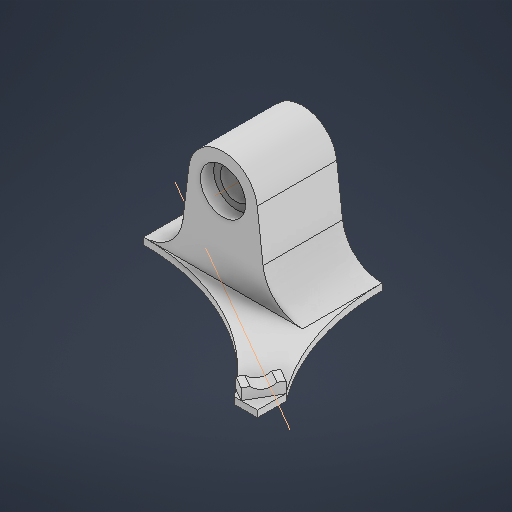
# Autodesk Inventor part: Support
Saved by Autodesk Inventor 2025.3 (Build 293356030, 356C)
## iProperties
Created: 2025-09-22
Part Number: Support
Material: Generic
Document SubType Name: Modeling
Designer: yo
Density: 1 g/cm^3
Appearance: Default
Author: yo
Autodesk Inventor part; units mm, degrees
ref_plane "YZ Plane" through (0, 0, 0) normal (1, 0, 0) x (0, 1, 0)
ref_plane "XZ Plane" through (0, 0, 0) normal (0, 1, 0) x (-1, 0, 0)
sketch "Sketch1" plane through (0, 0, 0) normal (0, 0, 1) x (1, 0, 0)
  circle A0 centre (0, 30) radius 8.525
  circle A1 centre (0, 30) radius 6
  arc A2 (-30, 0) -> (-15.1068, 13.2135) centre (-30, 15) ccw
  arc A3 (15.1068, 13.2135) -> (30, 0) centre (30, 15) ccw
  arc A4 (12.9075, 31.5483) -> (-12.9075, 31.5483) centre (0, 30) ccw
  line L0 (-12.9075, 31.5483) -> (-15.1068, 13.2135)
  line L1 (12.9075, 31.5483) -> (15.1068, 13.2135)
  line L2 (30, 0) -> (-30, 0)
  line L3 (-30, 0) -> (-30, -2.5)
  line L4 (-30, -2.5) -> (30, -2.5)
  line L5 (30, -2.5) -> (30, 0)
  point P0 (0, 0)
  point P1 (0, 0)
  dimension "d2" = 17.05
  dimension "d3" = 12
  dimension "d9" = 30
  dimension "d12" = 13
  dimension "d15" = 15
  dimension "d16" = 60
  dimension "d17" = 2.5
  constraints: 12 end point, 6 point on circle, 5 centre point, 5 tangent, 3 coincident, 2 horizontal alignment, 2 perpendicular, 2 vertical alignment, 1 equal length, 1 equal radius, 1 horizontal, 1 midpoint, 1 vertical
  measures "d2" diameter of A0
  measures "d3" diameter of A1
  measures "d9" distance of point (0, 0) A0.centre
  measures "d12" radius of A4
  measures "d15" radius of A2
  measures "d16" distance of L3.end L4.end
  measures "d17" distance of L2.end L3.end
extrude "Extrusion3" add sketch "Sketch1" along normal mid plane 30 contours A2 L0 A4 L1 A3 L2
extrude "Extrusion4" add sketch "Sketch1" along normal mid plane 20 contours A0
extrude "Extrusion5" add sketch "Sketch1" against normal blind 15 contours L2 L5 L4 L3
extrude "Extrusion6" add sketch "Sketch1" along normal blind 50 contours L2 L5 L4 L3
ref_plane "Work Plane1" through (30, -2.5, 50) normal (0.866, 0, 0.5) x (0, 1, 0)
ref_plane "Work Plane3" through (36.4952, -2.5, 53.75) normal (0.866, 0, 0.5) x (0, 1, 0)
sketch "Sketch5" plane through (36.4952, -2.5, 53.75) normal (0.866, 0, 0.5) x (0, 1, 0)
  line L0 (2.5, -30.3109) -> (2.5, -18.3109) construction
  circle A0 centre (10.5, -12.1087) radius 5.35
  circle A1 centre (10.5, -12.1087) radius 7.3 construction
  line L1 (2.5, -18.3109) -> (6.65, -18.3109)
  line L2 (6.65, -18.3109) -> (6.65, -5.9065)
  line L3 (6.65, -5.9065) -> (2.5, -5.9065)
  line L4 (2.5, -5.9065) -> (2.5, -18.3109)
  point P0 (6.65, -15.8235)
  point P1 (6.65, -8.3938)
  dimension "d46" = 12
  dimension "d47" = 10.7
  dimension "d48" = 14.6
  dimension "d49" = 8
  dimension "d51" = 1.5
  constraints: 10 end point, 2 centre point, 2 parallel, 2 point on circle, 1 coincident, 1 horizontal, 1 perpendicular, 1 vertical
  measures "d46" distance of L0.start L0.end
  measures "d47" diameter of A0
  measures "d48" diameter of A1
  measures "d49" distance from line of L4 A0.centre
  measures "d51" distance edge to line of A0 L2
extrude "Extrusion9" add sketch "Sketch5" along normal mid plane 5.5 contours A0 L2 L1 L4 L3
sketch "Sketch6" plane through (30, -2.5, -15) normal (1, 0, 0) x (0, 0, -1)
  line L0 (0, 0) -> (-65, 0) projected
  line L1 (0, 2.5) -> (0, 0) projected
  line L2 (0, 2.5) -> (-30, 2.5) projected
  line L3 (-30, 2.5) -> (-65, 2.5) projected
  line L4 (-65, 0) -> (-65, 2.5) projected
  point P0 (-15, 2.5)
extrude "Extrusion10" add sketch "Sketch6" along normal blind 18
sketch "Sketch7" plane through (-30, 0, 15) normal (0, 1, 0) x (1, 0, 0)
  line L0 (0, 30) -> (0, -35) projected
  arc A0 (69.1673, -35) -> (0, 0) centre (0, -85.8445) ccw
  line L1 (0, -35) -> (78, -35) projected
  line L2 (0, 0) -> (60, 0) projected
  arc A1 (60, 30) -> (78, -24.2242) centre (150.6739, 30) ccw
  line L3 (60, 30) -> (60, 0) projected
  line L4 (78, 30) -> (78, -35) projected
  line L5 (60, 30) -> (78, 30) projected
  point P0 (30, 15)
  point P1 (67.0668, -32.2599)
  point P2 (78.0322, -24.2673)
  constraints: 6 point on circle, 3 point on line, 2 centre point, 2 tangent
extrude "Extrusion11" cut sketch "Sketch7" against normal through all contours A0 L1 L0 | L5 L4 A1
body "Solid2"
